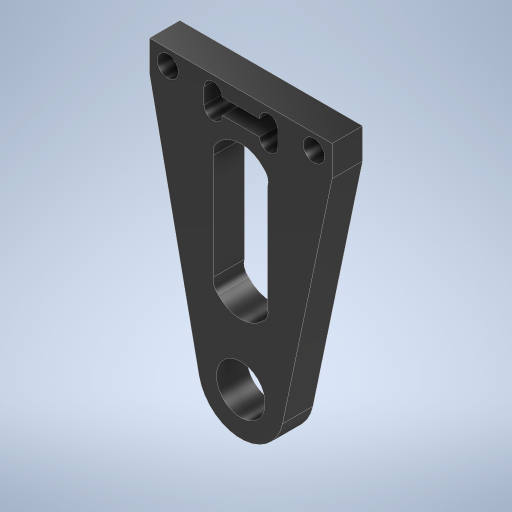
# Autodesk Inventor part: LegRollSliderFrame
Saved by Autodesk Inventor 2024.2 (Build 282272000, 272)
## iProperties
Created: 2024-01-04
Part Number: LegRollSliderFrame
Material: Aluminum 7075
Document SubType Name: Modeling
Designer: Masato Kubotera
Density: 2.81 g/cm^3
Appearance: Glossy - Black
Vendor: meviy
Mass: 10.3162 g
Surface Area: 28.8602 cm^2
Volume: 3.67124 cm^3
Author: Masato Kubotera
Autodesk Inventor part; units mm, degrees
ref_plane "YZ Plane" through (0, 0, 0) normal (1, 0, 0) x (0, 1, 0)
ref_plane "XZ Plane" through (0, 0, 0) normal (0, 1, 0) x (-1, 0, 0)
ref_plane "XY Plane" through (0, 0, 0) normal (0, 0, 1) x (1, 0, 0)
sketch "Sketch1" plane through (0, 0, 0) normal (1, 0, 0) x (0, 1, 0)
  line L0 (-15, 42.5) -> (15, 42.5)
  line L1 (15, 42.5) -> (15, 37.5)
  line L2 (15, 37.5) -> (6.8516, -1.434)
  arc A0 (-6.8516, -1.434) -> (6.8516, -1.434) centre (0, 0) ccw
  line L3 (0, 0) -> (0, 42.5) construction
  line L4 (-15, 42.5) -> (-15, 37.5)
  line L5 (-15, 37.5) -> (-6.8516, -1.434)
  line L6 (-15, 40) -> (15, 40) construction
  arc A1 (4.4, 32.3749) -> (-4.4, 32.3749) centre (0, 30) ccw
  line L7 (-4.4, 32.3749) -> (-4.4, 12.6251)
  line L8 (-4.4, 22.5) -> (4.4, 22.5) construction
  line L9 (4.4, 32.3749) -> (4.4, 12.6251)
  arc A2 (-4.4, 12.6251) -> (4.4, 12.6251) centre (0, 15) ccw
  circle A3 centre (0, 15) radius 15 construction
  line L10 (0, 0) -> (12.9904, 7.5) construction
  line L11 (12.9904, 7.5) -> (25.9808, 15) construction
  line L12 (6, 37.5) -> (-6, 37.5) construction
  line L13 (-6, 37.5) -> (-6, 40) construction
  line L14 (-6, 40) -> (6, 40) construction
  line L15 (6, 40) -> (6, 37.5) construction
  line L16 (6, 37.5) -> (-6, 40) construction
  line L17 (-6, 37.5) -> (6, 40) construction
  arc A4 (4.4, 31.1611) -> (3.6981, 33.3651) centre (2.4943, 31.768) ccw
  arc A5 (-3.6981, 33.3651) -> (-4.4, 31.1611) centre (-2.4943, 31.768) ccw
  arc A6 (3.6981, 11.6349) -> (4.4, 13.8389) centre (2.4943, 13.232) ccw
  arc A7 (-4.4, 13.8389) -> (-3.6981, 11.6349) centre (-2.4943, 13.232) ccw
  circle A8 centre (0, 0) radius 4 construction
  line L18 (6.05, 37.45) -> (-6.05, 37.45)
  line L19 (-6.05, 37.45) -> (-6.05, 40.05)
  line L20 (-6.05, 40.05) -> (6.05, 40.05)
  line L21 (6.05, 40.05) -> (6.05, 37.45)
  line L22 (6.05, 37.45) -> (-6.05, 40.05) construction
  line L23 (-6.05, 37.45) -> (6.05, 40.05) construction
  line L24 (-6.05, 38.75) -> (6.05, 38.75)
  arc A9 (6.05, 40.05) -> (3.05, 40.05) centre (4.55, 40.05) ccw
  arc A10 (3.05, 37.45) -> (6.05, 37.45) centre (4.55, 37.45) ccw
  arc A11 (-3.05, 40.05) -> (-6.05, 40.05) centre (-4.55, 40.05) ccw
  arc A12 (-6.05, 37.45) -> (-3.05, 37.45) centre (-4.55, 37.45) ccw
  circle A13 centre (0, 0) radius 30 construction
  point P0 (-12, 40)
  point P1 (12, 40)
  point P2 (0, 38.75)
  point P3 (-3.6981, 11.6349)
  point P4 (-4.4, 13.8389)
  point P5 (-4.4, 31.1611)
  point P6 (-3.6981, 33.3651)
  point P7 (4.4, 13.8389)
  point P8 (3.6981, 11.6349)
  point P9 (-3.05, 37.45)
  point P10 (-3.05, 40.05)
  point P11 (3.05, 37.45)
  dimension "d0" = 14
  dimension "d1" = 5
  dimension "d3" = 30
  dimension "d4" = 5
  dimension "d5" = 8.8
  dimension "d6" = 15
  dimension "d7" = 60
  dimension "d8" = 15
  dimension "d11" = 24
  dimension "d12" = 12
  dimension "d14" = 2
  dimension "d31" = 8
  dimension "d34" = 1.5
  dimension "d35" = 0.05
  dimension "d36" = 0.05
  dimension "d37" = 5
  dimension "d38" = 2.5
  dimension "d42" = 15
  dimension "d43" = 2.5
  constraints: 50 end point, 29 point on circle, 21 symmetric about line, 14 centre point, 11 midpoint, 8 point on line, 4 coincident, 4 horizontal, 4 parallel, 3 vertical, 2 perpendicular, 1 collinear, 1 tangent, 7 other
  measures "d0" diameter of A0
  measures "d1" distance of L0.end L1.end
  measures "d3" distance of L0.start L0.end
  measures "d4" radius of A1
  measures "d5" distance between parallel lines of L9 L7
  measures "d6" radius of A3
  measures "d7" angle of L3 L10
  measures "d8" distance of L10.end L11.end
  measures "d11" distance of point (12, 40) point (-12, 40)
  measures "d12" distance of L13.end L14.end
  measures "d14" radius of A4
  measures "d31" diameter of A8
  measures "d34" radius of A9
  measures "d35" distance between parallel lines of L14 L20
  measures "d36" distance between parallel lines of L15 L21
  measures "d37" distance between parallel lines of L12 L0
  measures "d38" distance between parallel lines of L14 L0
  measures "d42" distance of A2.centre A1.centre
  measures "d43" distance edge to line of A1 L12
extrude "Extrusion1" add sketch "Sketch1" along normal blind 5
hole "Hole1" at (0, -12, 40) at (0, 12, 40) direction (1, 0, 0) diameter 3.5 end through all
hole "Hole2" at (0, 0, 0) direction (1, 0, 0) diameter 8 end through all
equation "\"d36\" = d35"
equation "\"d42\" = d8"
equation "\"d24\" = d31"
body "Solid1"
